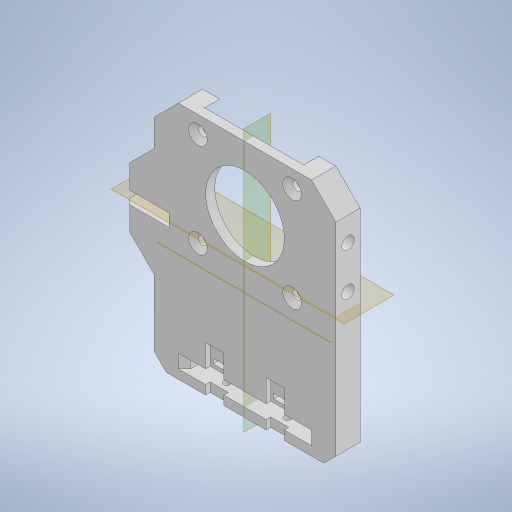
# Autodesk Inventor part: каретка
Saved by Autodesk Inventor 2023.1 (Build 271208000, 208)
## iProperties
Created: 2025-12-14
Part Number: каретка
Material: Типовые
Document SubType Name: Modeling
Designer: DELL
Density: 1 g/cm^3
Appearance: По умолчанию
Author: DELL
Autodesk Inventor part; units mm, degrees
ref_plane "YZ Plane" through (0, 0, 0) normal (1, 0, 0) x (0, 1, 0)
ref_plane "XZ Plane" through (0, 0, 0) normal (0, 1, 0) x (-1, 0, 0)
ref_plane "XY Plane" through (0, 0, 0) normal (0, 0, 1) x (1, 0, 0)
sketch "Эскиз1" plane through (0, 0, 0) normal (0, 0, 1) x (1, 0, 0)
  line L0 (16.9838, 20.6364) -> (20.6364, 16.9838) construction
  arc A0 (16.9838, 20.6364) -> (16.3474, 20.9) centre (16.3474, 20) ccw construction
  line L1 (-16.3474, 20.9) -> (16.3474, 20.9) construction
  arc A1 (-16.3474, 20.9) -> (-16.9838, 20.6364) centre (-16.3474, 20) ccw construction
  line L2 (-20.6364, 16.9838) -> (-16.9838, 20.6364) construction
  arc A2 (-20.6364, 16.9838) -> (-20.9, 16.3474) centre (-20, 16.3474) ccw construction
  line L3 (-20.9, -16.3474) -> (-20.9, 16.3474) construction
  arc A3 (-20.9, -16.3474) -> (-20.6364, -16.9838) centre (-20, -16.3474) ccw construction
  line L4 (-16.9838, -20.6364) -> (-20.6364, -16.9838) construction
  arc A4 (-16.9838, -20.6364) -> (-16.3474, -20.9) centre (-16.3474, -20) ccw construction
  line L5 (16.3474, -20.9) -> (-16.3474, -20.9) construction
  arc A5 (16.3474, -20.9) -> (16.9838, -20.6364) centre (16.3474, -20) ccw construction
  line L6 (20.6364, -16.9838) -> (16.9838, -20.6364) construction
  arc A6 (20.6364, -16.9838) -> (20.9, -16.3474) centre (20, -16.3474) ccw construction
  line L7 (20.9, 16.3474) -> (20.9, -16.3474) construction
  arc A7 (20.9, 16.3474) -> (20.6364, 16.9838) centre (20, 16.3474) ccw construction
  circle A8 centre (15.5574, -15.5574) radius 1.45 construction
  circle A9 centre (0, 0) radius 11 construction
  circle A10 centre (-15.5574, -15.5574) radius 1.45 construction
  circle A11 centre (-15.5574, 15.5574) radius 1.45 construction
  circle A12 centre (15.5574, 15.5574) radius 1.45 construction
  circle A13 centre (0, 0) radius 11 construction
  circle A14 centre (15.5574, 15.5574) radius 1.45
  circle A15 centre (-15.5574, 15.5574) radius 1.45
  circle A16 centre (15.5574, -15.5574) radius 1.45
  circle A17 centre (-15.5574, -15.5574) radius 1.45
  arc A18 (17.2667, 20.9192) -> (16.3474, 21.3) centre (16.3474, 20) ccw
  line L8 (17.2667, 20.9192) -> (20.9192, 17.2667)
  arc A19 (21.3, 16.3474) -> (20.9192, 17.2667) centre (20, 16.3474) ccw
  line L9 (21.3, 16.3474) -> (21.3, -16.3474)
  arc A20 (20.9192, -17.2667) -> (21.3, -16.3474) centre (20, -16.3474) ccw
  line L10 (20.9192, -17.2667) -> (17.2667, -20.9192)
  arc A21 (16.3474, -21.3) -> (17.2667, -20.9192) centre (16.3474, -20) ccw
  line L11 (16.3474, -21.3) -> (-16.3474, -21.3)
  arc A22 (-17.2667, -20.9192) -> (-16.3474, -21.3) centre (-16.3474, -20) ccw
  line L12 (-17.2667, -20.9192) -> (-20.9192, -17.2667)
  arc A23 (-21.3, -16.3474) -> (-20.9192, -17.2667) centre (-20, -16.3474) ccw
  line L13 (-21.3, -16.3474) -> (-21.3, 16.3474)
  arc A24 (-20.9192, 17.2667) -> (-21.3, 16.3474) centre (-20, 16.3474) ccw
  line L14 (-20.9192, 17.2667) -> (-17.2667, 20.9192)
  arc A25 (-16.3474, 21.3) -> (-17.2667, 20.9192) centre (-16.3474, 20) ccw
  line L15 (-16.3474, 21.3) -> (16.3474, 21.3)
  circle A26 centre (0, 0) radius 13
  point P0 (0, 0)
  dimension "d196" = 0.4
  dimension "d242" = 2
  constraints: 16 end point, 16 point on circle, 14 centre point, 5 coincident, 5 concentric, 15 other
  measures "d196" distance between parallel lines of L1 L15
  measures "d242" radial gap between concentric circles of A9 A26
extrude "Выдавливание1" add sketch "Эскиз1" along normal blind 3
sketch "Эскиз2" plane through (0, 0, 3) normal (0, 0, 1) x (1, 0, 0)
  line L0 (-30, -22.7) -> (30, -22.7)
  line L1 (30, -22.7) -> (30, 21.3)
  line L2 (30, 21.3) -> (-30, 21.3)
  line L3 (-30, 21.3) -> (-30, -22.7)
  line L4 (-30, -22.7) -> (30, -22.7)
  line L5 (30, -22.7) -> (30, -57.7)
  line L6 (30, -57.7) -> (-30, -57.7)
  line L7 (-30, -57.7) -> (-30, -22.7)
  arc A0 (-16.9838, -20.6364) -> (-16.3474, -20.9) centre (-16.3474, -20) ccw
  line L8 (-16.3474, -20.9) -> (16.3474, -20.9)
  arc A1 (16.3474, -20.9) -> (16.9838, -20.6364) centre (16.3474, -20) ccw
  line L9 (20.9192, 17.2667) -> (17.2667, 20.9192) projected
  arc A2 (17.2667, 20.9192) -> (16.3474, 21.3) centre (16.3474, 20) ccw projected
  line L10 (16.3474, 21.3) -> (-16.3474, 21.3) projected
  arc A3 (-16.3474, 21.3) -> (-17.2667, 20.9192) centre (-16.3474, 20) ccw projected
  line L11 (-17.2667, 20.9192) -> (-20.9192, 17.2667) projected
  arc A4 (-20.9192, 17.2667) -> (-21.3, 16.3474) centre (-20, 16.3474) ccw projected
  line L12 (-21.3, 16.3474) -> (-21.3, -16.3474) projected
  arc A5 (-21.3, -16.3474) -> (-20.9192, -17.2667) centre (-20, -16.3474) ccw projected
  line L13 (-20.9192, -17.2667) -> (-17.2667, -20.9192) projected
  arc A6 (-17.2667, -20.9192) -> (-16.3474, -21.3) centre (-16.3474, -20) ccw projected
  line L14 (-16.3474, -21.3) -> (16.3474, -21.3) projected
  arc A7 (16.3474, -21.3) -> (17.2667, -20.9192) centre (16.3474, -20) ccw projected
  line L15 (17.2667, -20.9192) -> (20.9192, -17.2667) projected
  arc A8 (20.9192, -17.2667) -> (21.3, -16.3474) centre (20, -16.3474) ccw projected
  line L16 (21.3, -16.3474) -> (21.3, 16.3474) projected
  arc A9 (21.3, 16.3474) -> (20.9192, 17.2667) centre (20, 16.3474) ccw projected
  circle A10 centre (-15.5574, -15.5574) radius 1.45 projected
  circle A11 centre (15.5574, -15.5574) radius 1.45 projected
  circle A12 centre (-15.5574, 15.5574) radius 1.45 projected
  circle A13 centre (15.5574, 15.5574) radius 1.45 projected
  point P0 (0, 21.3)
  point P1 (30, -22.7)
  dimension "d200" = -36
  dimension "d4" = 60
  dimension "d5" = 60
  dimension "d6" = 35
  dimension "d238" = 44
  constraints: 16 end point, 4 parallel, 2 centre point, 2 horizontal, 2 midpoint, 2 perpendicular
  measures "d4" distance of L2.end L1.end
  measures "d5" distance of L5.end L6.end
  measures "d6" distance of L4.end L5.end
  measures "d238" distance of L0.end L1.end
extrude "Выдавливание2" add sketch "Эскиз2" against normal blind 8 contours L3 L2 A3 L11 A4 L12 A5 L13 A6 L14 A7 L15 A8 L16 A9 L9 A2 L1 L0 | L0 L5 L6 L7
ref_plane "РабПлоскость4" through (-23, -29.9, -1) normal (0, -1, 0) x (1, 0, 0)
chamfer "Фаска1" distance 4 angle 45 2 edges at (30, -57.7, -1) (-30, -57.7, -1)
chamfer "Фаска2" distance 8 angle 45 2 edges at (30, 21.3, -1) (-30, 21.3, -1)
sketch "Эскиз25" plane through (0, 0, 3) normal (0, 0, 1) x (1, 0, 0)
  line L0 (-20, -50.2) -> (20, -50.2)
  line L1 (20, -50.2) -> (20, -54.7)
  line L2 (20, -54.7) -> (-20, -54.7)
  line L3 (-20, -54.7) -> (-20, -50.2)
  line L4 (-20, -50.2) -> (20, -54.7) construction
  line L5 (20, -50.2) -> (-20, -54.7) construction
  line L6 (-26, -57.7) -> (26, -57.7) construction
  line L7 (26, -57.7) -> (-26, -57.7) projected
  line L8 (0, -57.7) -> (0, 21.1) construction
  point P0 (0, 0)
  point P1 (0, -52.45)
  dimension "d170" = 40
  dimension "d171" = 4.5
  dimension "d172" = 3
  constraints: 14 end point, 3 midpoint, 2 parallel, 1 horizontal, 1 perpendicular, 1 point on line
  measures "d170" distance of L1.end L2.end
  measures "d171" distance of L0.end L1.end
  measures "d172" distance between parallel lines of L6 L2
extrude "Выдавливание25" cut sketch "Эскиз25" against normal blind 8
sketch "Эскиз27" plane through (-26, -57.7, 3) normal (0, -1, 0) x (1, 0, 0)
  line L0 (0, -8) -> (0, 0) construction
  line L1 (52, 0) -> (52, -8) construction
  line L2 (0, -4) -> (52, -4) construction
  circle A0 centre (16, -4) radius 1.1
  line L3 (46, 0) -> (46, -8) construction
  line L4 (6, 0) -> (46, 0) construction
  line L5 (46, 0) -> (46, -8) construction
  line L6 (46, -8) -> (6, -8) construction
  line L7 (6, -8) -> (6, 0) construction
  line L8 (6, 0) -> (46, -8) construction
  line L9 (46, 0) -> (6, -8) construction
  circle A1 centre (36, -4) radius 1.1
  point P0 (26, -4)
  dimension "d177" = 2.2
  dimension "d178" = 10
  dimension "d179" = 2.2
  dimension "d180" = 10
  constraints: 14 end point, 5 midpoint, 2 centre point, 2 parallel, 2 point on line, 1 horizontal, 1 perpendicular
  measures "d177" diameter of A0
  measures "d178" distance from line of L7 A0.centre
  measures "d179" diameter of A1
  measures "d180" distance from line of L3 A1.centre
extrude "Выдавливание26" cut sketch "Эскиз27" against normal blind 14
sketch "Эскиз28" plane through (0, 0, 3) normal (0, 0, 1) x (1, 0, 0)
  line L0 (20, -54.7) -> (-20, -54.7) construction
  line L1 (-20, -54.7) -> (-20, -50.2) construction
  line L2 (-20, -50.2) -> (20, -50.2) construction
  line L3 (20, -50.2) -> (20, -54.7) construction
  line L4 (-26, -57.7) -> (26, -57.7) projected
  line L5 (-13, -57.7) -> (-7, -57.7)
  line L6 (-7, -57.7) -> (-7, -42.7)
  line L7 (-7, -42.7) -> (-13, -42.7)
  line L8 (-13, -42.7) -> (-13, -57.7)
  line L9 (-10, -42.7) -> (-10, -57.7) construction
  point P0 (0, 0)
  point P1 (-10, -50.2)
  point P2 (-20, -52.45)
  point P3 (-7, -57.7)
  point P4 (-7, -57.8225)
  dimension "d183" = 6
  dimension "d184" = 15
  dimension "d185" = 10
  constraints: 10 end point, 4 midpoint, 2 parallel, 1 horizontal, 1 perpendicular, 1 point on line
  measures "d183" distance of L7.end L6.end
  measures "d184" distance of L6.end L5.end
  measures "d185" horizontal distance of point (-10, -50.2) point (-20, -52.45)
extrude "Выдавливание27" cut sketch "Эскиз28" against normal blind 1.5
ref_plane "РабПлоскость8" through (0, 0, -1) normal (0, 0, -1) x (-1, 0, 0)
mirror "Зеркальное отражение4" about plane through (0, 0, 0) normal (1, 0, 0) of "Выдавливание27"
mirror "Зеркальное отражение5" about plane through (0, 0, -1) normal (0, 0, -1) of "Выдавливание27", "Зеркальное отражение4"
sketch "Эскиз29" plane through (0, 0, 1.5) normal (0, 0, 1) x (1, 0, 0)
  line L0 (-13, -42.7) -> (-7, -42.7) construction
  line L1 (-13, -50.2) -> (-13, -42.7) construction
  line L2 (7, -50.2) -> (7, -42.7) construction
  line L3 (7, -42.7) -> (13, -42.7) construction
  line L4 (-13, -42.7) -> (-7, -42.7) projected
  line L5 (-10, -42.7) -> (-10, -42.7) construction
  line L6 (-12, -47.4) -> (-8, -47.4)
  line L7 (-8, -47.4) -> (-8, -49)
  line L8 (-8, -49) -> (-12, -49)
  line L9 (-12, -49) -> (-12, -47.4)
  line L10 (-12, -47.4) -> (-8, -49) construction
  line L11 (-8, -47.4) -> (-12, -49) construction
  line L12 (-13, -50.2) -> (-7, -50.2) projected
  line L13 (7, -57.7) -> (-7, -57.7) construction
  line L14 (0, -57.7) -> (0, -38.1038) construction
  line L15 (12, -47.4) -> (8, -47.4)
  line L16 (8, -47.4) -> (8, -49)
  line L17 (8, -49) -> (12, -49)
  line L18 (12, -49) -> (12, -47.4)
  point P0 (0, 0)
  point P1 (-10, -48.2)
  dimension "d188" = 4
  dimension "d189" = 1.6
  dimension "d190" = 1.2
  constraints: 24 end point, 4 midpoint, 4 symmetric about line, 2 parallel, 2 vertical, 1 horizontal, 1 perpendicular, 1 point on line, 1 other
  measures "d188" distance of L7.end L8.end
  measures "d189" distance of L6.end L7.end
extrude "Выдавливание28" cut sketch "Эскиз29" against normal blind 10
chamfer "Фаска4" distance 2 angle 45 4 edges at (-20, -52.45, 3) (-20, -52.45, -5) (20, -52.45, 3) (20, -52.45, -5)
chamfer "Фаска5" distance 1.65 angle 45 4 edges at (-17.0074, 15.5574, 3) (-17.0074, -15.5574, 3) (14.1074, 15.5574, 3) (14.1074, -15.5574, 3)
ref_plane "РабПлоскость9" through (0, -53.7, -5) normal (-1, 0, 0) x (0, 0, 1)
ref_plane "РабПлоскость10" through (26, -21.7, -5) normal (0, -1, 0) x (1, 0, 0)
sketch "Эскиз30" plane through (26, -21.7, -5) normal (0, -1, 0) x (1, 0, 0)
  line L0 (-56, 0) -> (-56, 8) construction
  line L1 (-56, 8) -> (4, 8) construction
  line L2 (4, 8) -> (4, 0) construction
  line L3 (4, 0) -> (-56, 0) construction
  line L4 (-56, 8) -> (-66, 8)
  line L5 (-66, 8) -> (-66, -10)
  line L6 (-66, -10) -> (-56, -10)
  line L7 (-56, -10) -> (-56, 8)
  point P0 (-26, 5)
  point P1 (-46.0806, 0)
  point P2 (-5.9194, 0)
  dimension "d205" = 10
  dimension "d206" = 18
  constraints: 8 end point, 2 parallel, 1 horizontal, 1 perpendicular
  measures "d205" distance of L6.end L5.end
  measures "d206" distance of L5.end L4.end
extrude "Выдавливание29" add sketch "Эскиз30" against normal blind 16
ref_plane "РабПлоскость11" through (26, -13.7, -5) normal (0, 1, 0) x (1, 0, 0)
sketch "Эскиз31" plane through (26, -13.7, -5) normal (0, 1, 0) x (1, 0, 0)
  line L0 (-66, 10) -> (-66, -8) projected
  line L1 (-66, 10) -> (-66, -8) projected
  line L2 (-66, -8) -> (-56, -8) projected
  line L3 (-56, 0) -> (-56, -8) projected
  line L4 (-56, 0) -> (-56, 10) projected
  line L5 (-56, 10) -> (-66, 10) projected
  point P0 (-26, -5)
extrude "Выдавливание30" cut sketch "Эскиз31" along normal mid plane 4.2
chamfer "Фаска7" distance 10 angle 45 1 edges at (-30, -5.7, -1)
chamfer "Фаска8" distance 10 angle 45 1 edges at (-30, -21.7, -1)
sketch "Эскиз32" plane through (26, -21.7, -5) normal (0, -1, 0) x (1, 0, 0)
  line L0 (-56, -10) -> (-66, -10) construction
  line L1 (-66, -10) -> (-66, 0) construction
  circle A0 centre (-61, -6) radius 1.6
  point P0 (-26, 5)
  dimension "d220" = 3.2
  dimension "d223" = 4
  constraints: 1 centre point
  measures "d220" diameter of A0
  measures "d223" distance from line of L0 A0.centre
extrude "Выдавливание31" cut sketch "Эскиз32" against normal blind 16
chamfer "Фаска9" distance 5 distance2 10 1 edges at (-30, -8.65, -5) measured on face at (-29.5, -8.65, -5)
chamfer "Фаска10" distance 5 distance2 10 1 edges at (-30, -18.75, -5) measured on face at (-29.5, -18.75, -5)
chamfer "Фаска11" distance 2 angle 45 2 edges at (-40, -8.65, -15) (-40, -18.75, -15)
chamfer "Фаска12" distance 2 angle 45 4 edges at (-40, -8.65, 3) (-39.9999, -5.7, 3) (-40, -18.75, 3) (-39.9999, -21.7, 3)
sketch "Эскиз33" plane through (0, 0, -5) normal (0, 0, -1) x (-1, 0, 0)
  line L0 (25, -5.7) -> (25, -11.6) projected
  line L1 (30, -15.8) -> (38, -15.8) projected
  line L2 (25, -11.6) -> (30, -11.6)
  line L3 (30, -11.6) -> (30, -15.8)
  line L4 (30, -15.8) -> (25, -15.8)
  line L5 (25, -15.8) -> (25, -11.6)
  point P0 (0, 0)
  constraints: 8 end point, 2 parallel, 1 horizontal, 1 perpendicular
extrude "Выдавливание32" cut sketch "Эскиз33" against normal blind 8
sketch "Эскиз34" plane through (26, -5.7, -5) normal (0, 1, 0) x (1, 0, 0)
  circle A0 centre (-61, 6) radius 1.6 projected
  line L0 (-59.3257, 8.9) -> (-57.6514, 6)
  line L1 (-57.6514, 6) -> (-59.3257, 3.1)
  line L2 (-59.3257, 3.1) -> (-62.6743, 3.1)
  line L3 (-62.6743, 3.1) -> (-64.3486, 6)
  line L4 (-64.3486, 6) -> (-62.6743, 8.9)
  line L5 (-62.6743, 8.9) -> (-59.3257, 8.9)
  line L6 (-56, 10) -> (-64, 10) projected
  point P0 (-26, -5)
  dimension "d239" = 5.8
  constraints: 12 end point, 1 coincident, 1 parallel, 13 other
  measures "d239" distance between parallel lines of L5 L2
extrude "Выдавливание33" cut sketch "Эскиз34" against normal blind 2.4
sketch "Эскиз35" plane through (30, -53.7, 3) normal (1, 0, 0) x (0, 0, -1)
  circle A0 centre (4, 59) radius 1.6 construction
  circle A1 centre (4, 45) radius 1.6 construction
  circle A2 centre (4, 59) radius 2.1
  circle A3 centre (4, 45) radius 2.1
  point P0 (3, 53.7)
  dimension "d243" = 4.2
  dimension "d244" = 4.2
  constraints: 2 centre point, 2 coincident
  measures "d243" diameter of A2
  measures "d244" diameter of A3
extrude "Выдавливание34" cut sketch "Эскиз35" against normal blind 5
sketch "Эскиз36" plane through (0, 0, -5) normal (0, 0, -1) x (-1, 0, 0)
  circle A0 centre (-22, -27.3) radius 2.1
  line L0 (-30, 13.3) -> (-30, -53.7) projected
  line L1 (16.3474, -21.3) -> (-16.3474, -21.3) projected
  circle A1 centre (18, -27.3) radius 2.1
  point P0 (0, 0)
  dimension "d247" = 4.2
  dimension "d248" = 8
  dimension "d249" = 6
  dimension "d250" = 4.2
  dimension "d251" = 40
  constraints: 2 centre point
  measures "d247" diameter of A0
  measures "d248" distance from line of L0 A0.centre
  measures "d249" distance from line of L1 A0.centre
  measures "d250" diameter of A1
  measures "d251" distance of A0.centre A1.centre
extrude "Выдавливание35" cut sketch "Эскиз36" against normal blind 5
